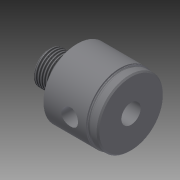
# Autodesk Inventor part: 17R000-0_rod_guide
Saved by Autodesk Inventor 2014 (Build 180170000, 170)
## iProperties
Category: PARTsolutions
Company: BIMBA
Created: 2014-01-18
Part Number: 17R000-0_rod_guide
Material: Generic
Catalog Web Link: www.cadenas.de
Description: Rod Guide-Original Line - Standard Air Cylinders
Vendor: BIMBA
Document SubType Name: Standard Catalog Part
Designer: Andrew Toennies
Manufacturer: BIMBA
Density: 1 g/cm^3
Appearance: RGB(211.00000262260440,211.00000262260440,211.00000262260440)
PSOL_IDENT_0: {$CADENAS_DATA\23d-libs\bimba\bimba\bimba_imperial\bimba_full_line\original_line_cylinders\standard_
PSOL_IDENT_1: air_cylinders\rod_guide.prj},232 {VTYP=3D},{NB=17R000-0_rod_guide},{LINA=17R000-0_rod_guide},{NN=Rod
PSOL_IDENT_2: Guide},{DATE=05.09.2013 09:10:53},{GEOMDATE=05.09.2013 11:10:00},{VERSION=},{LINEID=80},{LINESUBID=
PSOL_IDENT_3: -1},{WBVAR=MNT,ACTING,NR,K,Q,T1,T2,T3,T4,MB,TRIM,CUSH,RODTRANS}  {NB=17R000-0_rod_guide},{LINA=17R00
PSOL_IDENT_4: 0-0_rod_guide},{KT=DUMMY},{PN=17R000},{BORE=1.50000000},{BOREPN=17},{MNT=},{MNTALG='' , 'Front Nose'
PSOL_IDENT_5: , 'BF' , 'Front Block' , 'BFT' , 'Front Trunnion' , 'A' , 'Adjustable Stroke','BR' , 'Rear Block'},
PSOL_IDENT_6: {ACTING=R},{ACTINGALG= '' , 'Single Acting' , 'R' , 'Reverse/Double Acting' },{NR=},{NRALG= '' , 'Wi
PSOL_IDENT_7: thout Non-rotating Rod' , 'NR' , 'With Non-rotating Rod' },{K=},{Q=},{QALG= '' , 'Without Side Porte
PSOL_IDENT_8: d Rear Head' , 'Q' , 'With Side Ported Rear Head' },{T1=},{T2=},{T3=},{T4=},{MB=0},{A1=1.8750},{A1N=
PSOL_IDENT_9: 1.3120},{A1P=1.8750},{A1B=2.3750},{A2=0.6250},{A2N=0.6250},{A2P=0.6250},{A3=1.0000},{A3N=0.1880},{A3
PSOL_IDENT_10: P=1.0000},{A4=0.2525},{A4N=0.5000},{A4P=0.2525},{A5=0.0400},{A6=0.0000},{A6N=0.2500},{A6P=0.0000},{A
PSOL_IDENT_11: 7=0.2500},{A7N=0.6430},{A7P=0.2500},{A8=0.0300},{A8N=0.0300},{A8NR=0.0300},{D1=1.5565},{D1N=1.5565},
PSOL_IDENT_12: {D1P=1.5565},{D1B=1.5800},{D2=1.5115},{D3=0.0000},{D3N=0.8120},{D3P=0.0000},{D4=0.9690},{D4N=0.4730}
PSOL_IDENT_13: ,{D4P=0.9690},{D4NR=0.4395},{D5=0.4420},{D5N=0.4420},{D5NR=0.4395},{C1=0.030},{C2=0.0300},{C2N=0.030
PSOL_IDENT_14: 0},{C2P=0.0300},{C3=0.0000},{C3N=0.0000},{C3P=0.0000},{C4=0.0300},{C4N=0.0000},{C4P=0.0300},{NDM=0.7
PSOL_IDENT_15: 500},{NDMN=0.7500},{NDMP=0.7500},{TAB=UNF},{D6=0.7475},{D6N=0.7475},{D6P=0.7475},{A9=0.0940},{A9N=0.
PSOL_IDENT_16: 0940},{A9P=0.0940},{D7=0.6535},{D7N=0.6535},{D7P=0.6535},{A10=0.0965},{A10N=0.0965},{A10P=0.0965},{R
PSOL_IDENT_17: 1=0.0440},{R1N=0.0440},{R1P=0.0440},{D8=0.8120},{D9=0.7500},{D10=0.6880},{A11=0.8650},{A12=0.9590},{
PSOL_IDENT_18: A13=1.1150},{A14=0.6250},{A14N=0.6250},{A14B=0.7190},{D11=0.2500},{D11N=0.2500},{NDM2=0.4050},{NDM2N=
PSOL_IDENT_19: 0.4050},{NDM2DP=0.4200},{THREAD=0},{HEX=0.4375},{HEXN=0.4375},{S1=1.7500},{B1=0.1275},{B2=1.0050},{B
PSOL_IDENT_20: 22=0.0000},{DB=0.0000},{B3=0.6200},{B4=1.1300},{X1=0.1230},{X2=0.9975},{NDM3=0.3125},{NDM4=0.2500},{
PSOL_IDENT_21: NDM4DP=0.4950},{DD=1.7500},{CB=0.3750},{CBDP=0.2500},{PORT=1},{XT=1.0610},{XTX=1.0610},{XT1=0.5000},
PSOL_IDENT_22: {XT2=0.3800},{NDMH=0.7500},{OD=1.5565},{ID=1.5115},{G=0.0000},{PNUT=0.5310},{TRIM=0},{C11=0.3965},{C
PSOL_IDENT_23: 22=0.5625},{C33=0.3050},{C44=0.6250},{C55=0.8750},{CD1=0.2650},{CD2=0.1980},{CD3=0.1345},{CNDM3=0.25
PSOL_IDENT_24: 00},{CTAB3=UNS},{CUSH=0},{XX=1.13000},{LCD=0.0000},{RODTRANS=0.00000}
CNS_NN: Rod Guide
CNS_NT: Original Line - Standard Air Cylinders
CNS_NB: 17R000-0_rod_guide
CNS_NBSYN: $PN.-$RODTRANS._rod_guide
CNS_LINA: 17R000-0_rod_guide
CNS_PN: 17R000
CNS_BORE: 1 1/2
CNS_BOREPN: 17
CNS_MNT: Front Nose
CNS_MNTALG: '' , 'Front Nose' , 'BF' , 'Front Block' , 'BFT' , 'Front Trunnion' , 'A' , 'Adjustable Stroke','BR' , 'Rear Block'
CNS_ACTING: Reverse/Double Acting
CNS_ACTINGALG: '' , 'Single Acting' , 'R' , 'Reverse/Double Acting'
CNS_NR: Without Non-rotating Rod
CNS_NRALG: '' , 'Without Non-rotating Rod' , 'NR' , 'With Non-rotating Rod'
CNS_K: Standard
CNS_Q: Without Side Ported Rear Head
CNS_QALG: '' , 'Without Side Ported Rear Head' , 'Q' , 'With Side Ported Rear Head'
CNS_T1: without T1
CNS_T2: without T2
CNS_T3: without T3
CNS_T4: without T4
CNS_MB: 0
CNS_A1: 1.8750
CNS_A1N: 1.3120
CNS_A1P: 1.8750
CNS_A1B: 2.3750
CNS_A2: 0.6250
CNS_A2N: 0.6250
CNS_A2P: 0.6250
CNS_A3: 1.0000
CNS_A3N: 0.1880
CNS_A3P: 1.0000
CNS_A4: 0.2525
CNS_A4N: 0.5000
CNS_A4P: 0.2525
CNS_A5: 0.0400
CNS_A6: 0.0000
CNS_A6N: 0.2500
CNS_A6P: 0.0000
CNS_A7: 0.2500
CNS_A7N: 0.6430
CNS_A7P: 0.2500
CNS_A8: 0.0300
CNS_A8N: 0.0300
CNS_A8NR: 0.0300
CNS_D1: 1.5565
CNS_D1N: 1.5565
CNS_D1P: 1.5565
CNS_D1B: 1.5800
CNS_D2: 1.5115
CNS_D3: 0.0000
CNS_D3N: 0.8120
CNS_D3P: 0.0000
CNS_D4: 0.9690
CNS_D4N: 0.4730
CNS_D4P: 0.9690
CNS_D4NR: 0.4395
CNS_D5: 0.4420
CNS_D5N: 0.4420
CNS_D5NR: 0.4395
CNS_C1: 0.030
CNS_C2: 0.0300
CNS_C2N: 0.0300
CNS_C2P: 0.0300
CNS_C3: 0.0000
CNS_C3N: 0.0000
CNS_C3P: 0.0000
CNS_C4: 0.0300
CNS_C4N: 0.0000
CNS_C4P: 0.0300
CNS_NDM: 0.7500
CNS_NDMN: 0.7500
CNS_NDMP: 0.7500
CNS_TAB: UNF
CNS_D6: 0.7475
CNS_D6N: 0.7475
CNS_D6P: 0.7475
CNS_A9: 0.0940
CNS_A9N: 0.0940
CNS_A9P: 0.0940
CNS_D7: 0.6535
CNS_D7N: 0.6535
CNS_D7P: 0.6535
CNS_A10: 0.0965
CNS_A10N: 0.0965
CNS_A10P: 0.0965
CNS_R1: 0.0440
CNS_R1N: 0.0440
CNS_R1P: 0.0440
CNS_D8: 0.8120
CNS_D9: 0.7500
CNS_D10: 0.6880
CNS_A11: 0.8650
CNS_A12: 0.9590
CNS_A13: 1.1150
CNS_A14: 0.6250
CNS_A14N: 0.6250
CNS_A14B: 0.7190
CNS_D11: 0.2500
CNS_D11N: 0.2500
CNS_NDM2: 0.4050
CNS_NDM2N: 0.4050
CNS_NDM2DP: 0.4200
CNS_THREAD: 0
CNS_HEX: 0.4375
CNS_HEXN: 0.4375
CNS_S1: 1.7500
CNS_B1: 0.1275
CNS_B2: 1.0050
CNS_B22: 0.0000
CNS_DB: 0.0000
CNS_B3: 0.6200
CNS_B4: 1.1300
CNS_X1: 0.1230
CNS_X2: 0.9975
CNS_NDM3: 0.3125
CNS_NDM4: 0.2500
CNS_NDM4DP: 0.4950
CNS_DD: 1.7500
CNS_CB: 0.3750
CNS_CBDP: 0.2500
CNS_PORT: 1
CNS_XT: 1.0610
CNS_XTX: 1.0610
CNS_XT1: 0.5000
CNS_XT2: 0.3800
CNS_NDMH: 0.7500
CNS_OD: 1.5565
CNS_ID: 1.5115
CNS_G: 0.0000
CNS_PNUT: 0.5310
CNS_TRIM: 0
CNS_C11: 0.3965
CNS_C22: 0.5625
CNS_C33: 0.3050
CNS_C44: 0.6250
CNS_C55: 0.8750
CNS_CD1: 0.2650
CNS_CD2: 0.1980
CNS_CD3: 0.1345
CNS_CNDM3: 0.2500
CNS_CTAB3: UNS
CNS_CUSH: 0
CNS_XX: 1.13000
CNS_LCD: 0.0000
CNS_RODTRANS: 0.00000
SUPPLIER: BIMBA
ARTICLENO: 17R000-0_rod_guide
BOMINFO: 17R000-0_rod_guide
CREATOR: CADENAS GmbH
Title: 17R000-0_rod_guide
Author: Cadenas PARTsolutions
Comments: Original Line - Standard Air Cylinders
Autodesk Inventor part; units mm, degrees
ref_plane "YZ Plane" through (0, 0, 0) normal (1, 0, 0) x (0, 1, 0)
ref_plane "XZ Plane" through (0, 0, 0) normal (0, 1, 0) x (-1, 0, 0)
ref_plane "XY Plane" through (0, 0, 0) normal (0, 0, 1) x (1, 0, 0)
sketch "Sketch_2" plane through (0, 0, 0) normal (0, 0, 1) x (1, 0, 0)
  line L0 (15.875, 0) -> (0, 0)
  line L1 (0, 0) -> (0, 8.589)
  line L2 (0, 8.589) -> (0.936, 9.525)
  line L3 (0.936, 9.525) -> (9.31, 9.525)
  line L4 (9.31, 9.525) -> (10.2623, 8.6108)
  arc A0 (10.2623, 8.6108) -> (11.0363, 8.2995) centre (11.0363, 9.417) ccw
  line L5 (11.0363, 8.2995) -> (12.3698, 8.2995)
  arc A1 (12.3698, 8.2995) -> (13.4874, 9.4171) centre (12.3698, 9.417) ccw
  line L6 (13.4874, 9.4171) -> (13.4874, 9.4933)
  line L7 (13.4874, 9.4933) -> (15.875, 9.4933)
  line L8 (15.875, 9.4933) -> (15.875, 0)
  line L9 (15.875, 0) -> (0, 0)
  constraints: 20 end point, 4 point on circle, 2 centre point
revolve "Revolution1" add sketch "Sketch_2" angle 360 about axis through (15.875, 0, 0) along (1, 0, 0)
thread "Thread1" size "3/4-16 UNF" class "2A" standard "ANSI Unified Screw Threads" full length
sketch "Sketch_3" plane through (0, 0, 0) normal (0, 0, 1) x (1, 0, 0)
  line L0 (47.625, 0) -> (15.875, 0)
  line L1 (15.875, 0) -> (15.875, 19.0055)
  line L2 (15.875, 19.0055) -> (16.637, 19.7675)
  line L3 (16.637, 19.7675) -> (41.2115, 19.7675)
  line L4 (41.2115, 19.7675) -> (41.2115, 18.1801)
  line L5 (41.2115, 18.1801) -> (42.2275, 18.1801)
  line L6 (42.2275, 18.1801) -> (43.2435, 19.196)
  line L7 (43.2435, 19.196) -> (46.863, 19.196)
  line L8 (46.863, 19.196) -> (47.625, 18.434)
  line L9 (47.625, 18.434) -> (47.625, 0)
  line L10 (47.625, 0) -> (15.875, 0)
  constraints: 22 end point
revolve "Revolution2" add sketch "Sketch_3" angle 360 about axis through (47.625, 0, 0) along (1, 0, 0)
sketch "Sketch3" plane through (0, 0, 0) normal (-1, 0, 0) x (0, 0, 1)
  point P0 (0, 0)
hole "Hole1" at (0, 0, 0) direction (1, 0, 0) diameter 11.2268 depth 47.625 countersink diameter 12.7508 countersink angle 90
sketch "Sketch_40" plane through (0, 0, 0) normal (0, 1, 0) x (-1, 0, 0)
  line L0 (-31.75, 19.7675) -> (-31.75, 0)
  line L1 (-31.75, 0) -> (-34.925, 0)
  line L2 (-34.925, 0) -> (-34.925, 7.7681)
  line L3 (-34.925, 7.7681) -> (-36.2564, 9.0996)
  line L4 (-36.2564, 9.0996) -> (-36.5895, 19.7675)
  line L5 (-36.5895, 19.7675) -> (-31.75, 19.7675)
  line L6 (-31.75, 19.7675) -> (-31.75, 0)
  constraints: 14 end point
revolve "Revolution3" cut sketch "Sketch_40" angle 360 about axis through (31.75, 0, 19.7675) along (0, 0, 1)
sketch "Sketch_47" plane through (0, 0, 0) normal (0, 0, 1) x (1, 0, 0)
  line L0 (42.2275, 0) -> (41.2115, 0)
  line L1 (41.2115, 17.9261) -> (42.2275, 17.9261)
  line L2 (42.2275, 17.9261) -> (42.2275, 18.1801)
  line L3 (42.2275, 18.1801) -> (41.7195, 18.1801)
  line L4 (41.7195, 18.1801) -> (41.3449, 18.5547)
  arc A0 (41.3449, 18.7343) -> (41.3449, 18.5547) centre (41.4347, 18.6445) ccw
  line L5 (41.3449, 18.7343) -> (42.294, 19.6834)
  line L6 (42.294, 19.6834) -> (42.294, 19.7675)
  line L7 (42.294, 19.7675) -> (42.0908, 19.7675)
  line L8 (42.0908, 19.7675) -> (41.2115, 18.8883)
  line L9 (41.2115, 18.8883) -> (41.2115, 17.9261)
  constraints: 20 end point, 2 point on circle, 1 centre point
revolve "Revolution4" add sketch "Sketch_47" angle 360 about axis through (42.2275, 0, 0) along (1, 0, 0)
ref_plane "dp1_XY" through (15.875, 9.4933, 0) normal (0, 0, 1) x (1, 0, 0)
ref_plane "dp1_YZ" through (15.875, 9.4933, 0) normal (1, 0, 0) x (0, 1, 0)
ref_plane "dp1_ZX" through (15.875, 9.4933, 0) normal (0, 1, 0) x (0, 0, 1)
ref_plane "dp2_XY" through (15.875, -9.4933, 0) normal (0, 0, 1) x (1, 0, 0)
ref_plane "dp2_YZ" through (15.875, -9.4933, 0) normal (1, 0, 0) x (0, 1, 0)
ref_plane "dp2_ZX" through (15.875, -9.4933, 0) normal (0, 1, 0) x (0, 0, 1)
ref_plane "port_XY" through (31.75, 0, 0) normal (0, 0, 1) x (1, 0, 0)
ref_plane "port_YZ" through (31.75, 0, 0) normal (1, 0, 0) x (0, 1, 0)
ref_plane "port_ZX" through (31.75, 0, 0) normal (0, 1, 0) x (0, 0, 1)
ref_plane "rod_guide_XY" through (0, 0, 0) normal (1, 0, 0) x (0, 0, -1)
ref_plane "rod_guide_YZ" through (0, 0, 0) normal (0, 0, -1) x (0, 1, 0)
ref_plane "rod_guide_ZX" through (0, 0, 0) normal (0, 1, 0) x (1, 0, 0)
ref_plane "s1_XY" through (13.4874, 0, 0) normal (0, 0, 1) x (1, 0, 0)
ref_plane "s1_YZ" through (13.4874, 0, 0) normal (1, 0, 0) x (0, 1, 0)
ref_plane "s1_ZX" through (13.4874, 0, 0) normal (0, 1, 0) x (0, 0, 1)
ref_plane "s2_XY" through (15.875, 0, 0) normal (0, 0, 1) x (1, 0, 0)
ref_plane "s2_YZ" through (15.875, 0, 0) normal (1, 0, 0) x (0, 1, 0)
ref_plane "s2_ZX" through (15.875, 0, 0) normal (0, 1, 0) x (0, 0, 1)
ref_plane "t1_XY" through (15.875, 0, 0) normal (1, 0, 0) x (0, 0, -1)
ref_plane "t1_YZ" through (15.875, 0, 0) normal (0, 0, -1) x (0, 1, 0)
ref_plane "t1_ZX" through (15.875, 0, 0) normal (0, 1, 0) x (1, 0, 0)
ref_plane "t111_XY" through (15.875, 0, 0) normal (1, 0, 0) x (0, 0, -1)
ref_plane "t111_YZ" through (15.875, 0, 0) normal (0, 0, -1) x (0, 1, 0)
ref_plane "t111_ZX" through (15.875, 0, 0) normal (0, 1, 0) x (1, 0, 0)
ref_plane "to_foot_bracket_XY" through (15.875, 0, 0) normal (1, 0, 0) x (0, 0, -1)
ref_plane "to_foot_bracket_YZ" through (15.875, 0, 0) normal (0, 0, -1) x (0, 1, 0)
ref_plane "to_foot_bracket_ZX" through (15.875, 0, 0) normal (0, 1, 0) x (1, 0, 0)
ref_plane "to_nut_XY" through (13.4874, 0, 0) normal (1, 0, 0) x (0, 0, -1)
ref_plane "to_nut_YZ" through (13.4874, 0, 0) normal (0, 0, -1) x (0, 1, 0)
ref_plane "to_nut_ZX" through (13.4874, 0, 0) normal (0, 1, 0) x (1, 0, 0)
ref_plane "to_rod_XY" through (0, 0, 0) normal (1, 0, 0) x (0, 0, -1)
ref_plane "to_rod_YZ" through (0, 0, 0) normal (0, 0, -1) x (0, 1, 0)
ref_plane "to_rod_ZX" through (0, 0, 0) normal (0, 1, 0) x (1, 0, 0)
ref_plane "to_screw_XY" through (31.75, 14.2875, -10.0711) normal (0, 1, 0) x (1, 0, 0)
ref_plane "to_screw_YZ" through (31.75, 14.2875, -10.0711) normal (1, 0, 0) x (0, 0, -1)
ref_plane "to_screw_ZX" through (31.75, 14.2875, -10.0711) normal (0, 0, -1) x (0, 1, 0)
ref_plane "to_trunnion_brackets_XY" through (26.9494, 0, 0) normal (0, 1, 0) x (1, 0, 0)
ref_plane "to_trunnion_brackets_YZ" through (26.9494, 0, 0) normal (1, 0, 0) x (0, 0, -1)
ref_plane "to_trunnion_brackets_ZX" through (26.9494, 0, 0) normal (0, 0, -1) x (0, 1, 0)
ref_plane "to_trunnion_brackets1_XY" through (26.9494, 22.225, 0) normal (0, 1, 0) x (1, 0, 0)
ref_plane "to_trunnion_brackets1_YZ" through (26.9494, 22.225, 0) normal (1, 0, 0) x (0, 0, -1)
ref_plane "to_trunnion_brackets1_ZX" through (26.9494, 22.225, 0) normal (0, 0, -1) x (0, 1, 0)
ref_plane "to_trunnion_brackets2_XY" through (26.9494, -22.225, 0) normal (0, 1, 0) x (1, 0, 0)
ref_plane "to_trunnion_brackets2_YZ" through (26.9494, -22.225, 0) normal (1, 0, 0) x (0, 0, -1)
ref_plane "to_trunnion_brackets2_ZX" through (26.9494, -22.225, 0) normal (0, 0, -1) x (0, 1, 0)
ref_plane "to_tube_XY" through (42.2275, 0, 0) normal (1, 0, 0) x (0, 0, -1)
ref_plane "to_tube_YZ" through (42.2275, 0, 0) normal (0, 0, -1) x (0, 1, 0)
ref_plane "to_tube_ZX" through (42.2275, 0, 0) normal (0, 1, 0) x (1, 0, 0)
body "Solid1"
